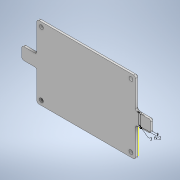
# Autodesk Inventor part: BatteryHolder
Saved by Autodesk Inventor 2022 (Build 260153000, 153)
## iProperties
Created: 2021-04-26
Part Number: BatteryHolder
Material: Generic
Document SubType Name: Modeling
Designer: lgnds
Density: 1 g/cm^3
Appearance: Default
Author: lgnds
Autodesk Inventor part; units mm, degrees
ref_plane "YZ Plane" through (0, 0, 0) normal (1, 0, 0) x (0, 1, 0)
ref_plane "XZ Plane" through (0, 0, 0) normal (0, 1, 0) x (-1, 0, 0)
ref_plane "XY Plane" through (0, 0, 0) normal (0, 0, 1) x (1, 0, 0)
sketch "Sketch1" plane through (0, 0, 0) normal (0, 0, 1) x (1, 0, 0)
  line L0 (-49, -36) -> (49, -36)
  line L1 (49, -36) -> (49, 36)
  line L2 (49, 36) -> (-49, 36)
  line L3 (-49, 36) -> (-49, -36)
  line L4 (-49, -36) -> (49, 36) construction
  line L5 (49, -36) -> (-49, 36) construction
  point P0 (0, 0)
  dimension "d0" = 98
  dimension "d1" = 72
  constraints: 12 end point, 2 midpoint, 2 parallel, 1 horizontal, 1 perpendicular
  measures "d0" distance of L1.end L2.end
  measures "d1" distance of L2.end L0.start
extrude "Extrusion1" add sketch "Sketch1" along normal blind 3
sketch "Sketch2" plane through (0, 0, 3) normal (0, 0, 1) x (1, 0, 0)
  circle A0 centre (-44.5, 31.5) radius 2
  line L0 (-68.6, 0) -> (68.6, 0) projected
  line L1 (0, 50.4) -> (0, -50.4) construction
  circle A1 centre (44.5, 31.5) radius 2
  circle A2 centre (-44.5, -31.5) radius 2
  circle A3 centre (44.5, -31.5) radius 2
  point P0 (0, 0)
  dimension "d4" = 4
  dimension "d5" = 89
  dimension "d6" = 63
  constraints: 4 centre point, 3 symmetric about line, 3 other
  measures "d4" diameter of A0
  measures "d5" distance of A1.centre A0.centre
  measures "d6" distance of A1.centre A3.centre
extrude "Extrusion2" cut sketch "Sketch2" against normal through all
sketch "Sketch3" plane through (0, 0, 3) normal (0, 0, 1) x (1, 0, 0)
  line L0 (-68.6, 0) -> (68.6, 0) construction
  line L1 (-64, -6) -> (-49, -6)
  line L2 (-49, -6) -> (-49, 6)
  line L3 (-49, 6) -> (-64, 6)
  line L4 (-64, 6) -> (-64, -6)
  line L5 (-64, -6) -> (-49, 6) construction
  line L6 (-49, -6) -> (-64, 6) construction
  line L7 (-49, 36) -> (-49, -36) construction
  line L8 (0, 50.4) -> (0, -50.4) projected
  line L9 (64, -6) -> (49, -6)
  line L10 (49, -6) -> (49, 6)
  line L11 (49, 6) -> (64, 6)
  line L12 (64, 6) -> (64, -6)
  line L13 (64, -6) -> (49, 6) construction
  line L14 (49, -6) -> (64, 6) construction
  point P0 (0, 0)
  point P1 (-56.5, 0)
  point P2 (-49, 0)
  point P3 (56.5, 0)
  point P4 (49, 0)
  dimension "d9" = 12
  dimension "d10" = 15
  constraints: 24 end point, 7 midpoint, 6 symmetric about line, 2 parallel, 1 horizontal, 1 perpendicular, 1 point on line
  measures "d9" distance between parallel lines of L3 L1
  measures "d10" distance between parallel lines of L2 L4
extrude "Extrusion3" add sketch "Sketch3" against normal up to surface (3 mm away)
fillet "Fillet1" radius 2 12 edges at (-49, 6, 1.5) (-49, -6, 1.5) (49, -6, 1.5) (49, 6, 1.5) (49, 36, 1.5) (-49, 36, 1.5) (-49, -36, 1.5) (-64, -6, 1.5) (-64, 6, 1.5) (49, -36, 1.5) (64, -6, 1.5) (64, 6, 1.5)
chamfer "Chamfer1" distance 1 angle 45 10 edges at (0, 36, 0) (-48.4142, 35.4142, 0) (-49, 21, 0) (-49, -21, 0) (-48.4142, -35.4142, 0) (0, -36, 0) (48.4142, -35.4142, 0) (49, -21, 0) (49, 21, 0) (48.4142, 35.4142, 0)
sketch "Sketch4" plane through (0, 0, 0) normal (0, 0, -1) x (-1, 0, 0)
  circle A0 centre (-51, -8) radius 1.5
  line L0 (-49, -8) -> (-49, -34) projected
  line L1 (-62, -6) -> (-51, -6) projected
  point P0 (0, 0)
  dimension "d17" = 2
  dimension "d18" = 2
  dimension "d19" = 3
  constraints: 1 centre point
  measures "d17" distance from line of L0 A0.centre
  measures "d18" distance from line of A0.centre L1
  measures "d19" diameter of A0
equation "\"d18\" = d17"
body "Solid1"
